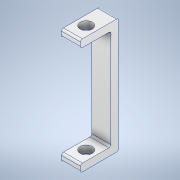
# Autodesk Inventor part: bobastacksupport
Saved by Autodesk Inventor 2022 (Build 260153000, 153)
## iProperties
Created: 2021-10-10
Part Number: bobastacksupport
Material: Aluminum 6061
Document SubType Name: Modeling
Designer: Bowen O'Steen
Density: 2.7 g/cm^3
Appearance: Aluminum - Flat
Author: Bowen O'Steen
Autodesk Inventor part; units mm, degrees
ref_plane "YZ Plane" through (0, 0, 0) normal (1, 0, 0) x (0, 1, 0)
ref_plane "XZ Plane" through (0, 0, 0) normal (0, 1, 0) x (-1, 0, 0)
ref_plane "XY Plane" through (0, 0, 0) normal (0, 0, 1) x (1, 0, 0)
sketch "Sketch1" plane through (0, 0, 0) normal (0, 0, 1) x (1, 0, 0)
  line L0 (-2.5, 15.2) -> (2.5, 15.2)
  line L1 (2.5, 15.2) -> (2.5, -15.2)
  line L2 (2.5, -15.2) -> (-2.5, -15.2)
  line L3 (-2.5, -15.2) -> (-2.5, 15.2)
  point P0 (0, 0)
  point P1 (2.5, 0)
  point P2 (0, 15.2)
  dimension "d0" = 30.4
  dimension "d1" = 5
  constraints: 8 end point, 2 midpoint, 2 parallel, 1 horizontal, 1 horizontal alignment, 1 perpendicular, 1 vertical alignment
  measures "d0" distance of L0.end L1.end
  measures "d1" distance of L0.start L0.end
extrude "Extrusion1" add sketch "Sketch1" along normal blind 2
sketch "Sketch2" plane through (-2.5, 15.2, 0) normal (0, 1, 0) x (1, 0, 0)
  line L0 (5, -2) -> (0, -2) projected
  line L1 (0, -2) -> (5, -2)
  line L2 (5, -2) -> (5, -10)
  line L3 (5, -10) -> (0, -10)
  line L4 (0, -10) -> (0, -2)
  point P0 (2.5, 0)
  dimension "d4" = 5
  dimension "d5" = 8
  constraints: 8 end point, 2 parallel, 1 horizontal, 1 perpendicular
  measures "d4" distance of L0.end L1.end
  measures "d5" distance of L3.end L0.end
extrude "Extrusion2" add sketch "Sketch2" against normal blind 2
mirror "Mirror1" about plane through (0, 0, 0) normal (0, 1, 0) of "Extrusion2"
sketch "Sketch3" plane through (-2.5, 15.2, 0) normal (0, 1, 0) x (1, 0, 0)
  line L0 (5, -10) -> (0, -10) projected
  line L1 (5, -2) -> (5, -10) projected
  line L2 (0, -2) -> (5, -2) projected
  line L3 (0, -10) -> (0, -2) projected
  point P0 (2.5, 0)
  point P1 (2.5, -6)
  point P2 (2.5, -2)
  point P3 (0, -6)
  constraints: 2 midpoint, 1 horizontal alignment, 1 vertical alignment
hole "Hole1" at (0, 15.2, 6) direction (0, -1, 0) diameter 3.2 depth 30.4 clearance for "Flat Head Machine Screw" size "M3" standard "Ansi Metric M Profile"
fillet "Fillet1" radius 0.5 8 edges at (0, 15.2, 0) (0, -15.2, 0) (0, -15.2, 10) (0, -13.2, 10) (0, -13.2, 2) (0, 13.2, 2) (0, 13.2, 10) (0, 15.2, 10)
body "Solid1"
